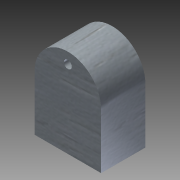
# Autodesk Inventor part: Rudder_Bracket
Saved by Autodesk Inventor 2011 SP1 (Build 150282100, 282)
## iProperties
Created: 2011-06-11
Part Number: Rudder_Bracket
Document SubType Name: Modeling
Designer: Andrew G. Meyer
Mass: 5.62513 g
Surface Area: 19.6015 cm^2
Volume: 5.62513 cm^3
Density: 1 g/cm^3
Author: Andrew G. Meyer
Autodesk Inventor part; units mm, degrees
ref_plane "YZ Plane" through (0, 0, 0) normal (1, 0, 0) x (0, 1, 0)
ref_plane "XZ Plane" through (0, 0, 0) normal (0, 1, 0) x (-1, 0, 0)
ref_plane "XY Plane" through (0, 0, 0) normal (0, 0, 1) x (1, 0, 0)
sketch "Sketch1" plane through (0, 0, 0) normal (0, 0, 1) x (1, 0, 0)
  line L0 (-9.525, 0) -> (9.525, 0)
  line L1 (9.525, 0) -> (9.525, 15.875)
  line L2 (-9.525, 0) -> (-9.525, 15.875)
  arc A0 (9.525, 15.875) -> (-9.525, 15.875) centre (0, 15.875) ccw
  point P0 (0, 0)
  dimension "d0" = 19.05
  dimension "d1" = 9.525
  dimension "d2" = 9.525
  dimension "d3" = 15.875
  constraints: 6 end point, 2 point on circle, 2 tangent, 1 centre point, 1 horizontal, 1 midpoint, 1 parallel, 1 perpendicular
  measures "d0" distance of L0.start L0.end
  measures "d1" distance from line of L2 point (0, 0)
  measures "d2" radius of A0
  measures "d3" distance of L0.end L1.end
extrude "Extrusion1" add sketch "Sketch1" along normal blind 12.7
hole "Hole1" at (0, 22.225, 12.7) direction (0, 0, -1) diameter 2.2606 depth 6.35
equation "\"d1\" = 0.5 * d0"
body "Solid1"
